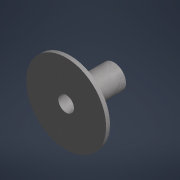
# Autodesk Inventor part: Tuerca3
Saved by Autodesk Inventor 2022 (Build 260153000, 153)
## iProperties
Created: 2021-09-20
Part Number: Tuerca3
Material: Steel, Alloy
Document SubType Name: Modeling
Designer: Andres
Density: 7.73 g/cm^3
Appearance: Semi-Polished
Author: Andres
Autodesk Inventor part; units mm, degrees
ref_plane "YZ Plane" through (0, 0, 0) normal (1, 0, 0) x (0, 1, 0)
ref_plane "XZ Plane" through (0, 0, 0) normal (0, 1, 0) x (-1, 0, 0)
ref_plane "XY Plane" through (0, 0, 0) normal (0, 0, 1) x (1, 0, 0)
sketch "Sketch1" plane through (0, 0, 0) normal (1, 0, 0) x (0, 1, 0)
  line L0 (0, -68.5665) -> (0, 42.4294) projected
  line L1 (0, 26.5728) -> (0, -52.7099)
  line L2 (-15, 8) -> (-15, -8)
  line L3 (-15, -8) -> (-12.5, -8)
  line L4 (-12.5, -8) -> (-12.5, -40)
  line L5 (-12.5, -40) -> (0, -40)
  line L6 (-15, 8) -> (-40, 8)
  line L7 (-40, 8) -> (-40, 16)
  line L8 (-40, 16) -> (0, 16)
  line L9 (-60, 0) -> (53.5817, 0) projected
  line L10 (-60, 10) -> (53.5817, 10) projected
  line L11 (-8, 16) -> (-8, -4)
  line L12 (-8, -4) -> (-10, -4)
  line L13 (-10, -4) -> (-10, -40)
  point P0 (0, 0)
  dimension "d1" = 80
  dimension "d2" = 8
  dimension "d3" = 8
  dimension "d4" = 25
  dimension "d5" = 30
  dimension "d8" = 20
  dimension "d11" = 16
  dimension "L_roscado" = 20
  dimension "d16" = 8
  dimension "d17" = 32
  constraints: 22 end point, 6 perpendicular, 6 point on line, 3 vertical, 1 horizontal
  measures "d1" diameter of L7 L1
  measures "d2" distance between parallel lines of L6 L9
  measures "d3" distance between parallel lines of L6 L8
  measures "d4" diameter of L4 L1
  measures "d5" diameter of L2 L1
  measures "d8" diameter of L13 L1
  measures "d11" diameter of L11 L1
  measures "L_roscado" distance between parallel lines of L8 L12
  measures "d16" distance between parallel lines of L9 L3
  measures "d17" distance between parallel lines of L3 L5
revolve "Revolution1" add sketch "Sketch1" angle 360 about axis through (0, 0, 26.5728) along (0, 0, -1) contours L5 L4 L3 L2 L9 L11 L12 L13 | L9 L2 L6 L7 L10 L11 | L10 L7 L8 L11
chamfer "Chamfer1" distance 8 angle 30 1 edges at (0, 15, 8) measured on face at (0, 15, 7.5)
chamfer "Chamfer2" distance 2 angle 45 1 edges at (0, 40, 8)
sketch "Sketch2" plane through (0, 0, 16) normal (0, 0, 1) x (1, 0, 0)
  circle A0 centre (0, 0) radius 32.5 construction
  point P0 (32.5, 0)
  point P1 (16.25, 28.1458)
  point P2 (-16.25, 28.1458)
  point P3 (-32.5, 0)
  point P4 (-16.25, -28.1458)
  point P5 (16.25, -28.1458)
  dimension "d24" = 65
  dimension "d27" = 360
  constraints: 2 horizontal alignment, 1 coincident, 9 other
hole "Hole1" at (32.5, 0, 16) at (16.25, 28.1458, 16) at (-16.25, 28.1458, 16) at (-32.5, 0, 16) at (-16.25, -28.1458, 16) at (16.25, -28.1458, 16) direction (0, 0, -1) diameter 3.4 end through all counterbore diameter 6.5 counterbore depth 3.4 clearance for "Socket Head Cap Screw ISO 4762" size "M3" standard "ISO"
sketch "Sketch3" plane through (0, 0, 16) normal (0, 0, 1) x (1, 0, 0)
  circle A0 centre (0, 0) radius 25
  circle A1 centre (0, 0) radius 8 projected
  dimension "d36" = 50
  constraints: 1 centre point, 1 coincident
  measures "d36" diameter of A0
extrude "Extrusion1" cut sketch "Sketch3" against normal blind 4
thread "Thread1" size "TR16x2" class "7H" standard "ISO Metric Trapezoidal Threads" full length
chamfer "Chamfer3" distance 2 angle 45 1 edges at (0, 10, -4)
chamfer "Chamfer4" distance 1 angle 45 1 edges at (-25, 0, 16)
chamfer "Chamfer5" distance 1 angle 45 1 edges at (0, 40, 16)
body "Solid1"
